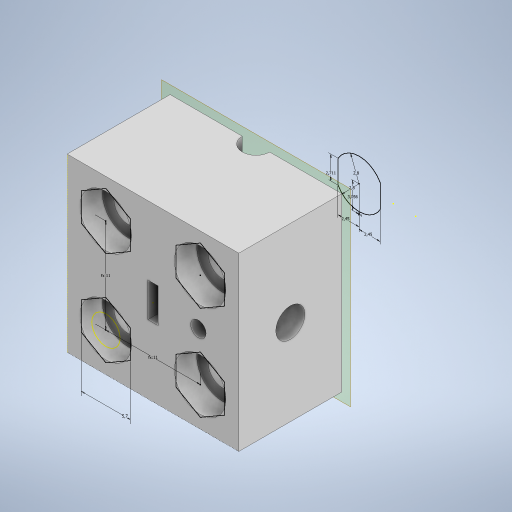
# Autodesk Inventor part: DFZ_bottom_fl_1mm_v3
Saved by Autodesk Inventor 2023 (Build 270158000, 158)
## iProperties
Created: 2019-07-31
Part Number: DFZ_bottom_fl_1mm_v3
Material: Generisch
Document SubType Name: Modeling
Designer: maximilian
Density: 1 g/cm^3
Appearance: Vorgabe
Author: maximilian
Autodesk Inventor part; units mm, degrees
ref_plane "YZ Plane" through (0, 0, 0) normal (1, 0, 0) x (0, 1, 0)
ref_plane "XZ Plane" through (0, 0, 0) normal (0, 1, 0) x (-1, 0, 0)
ref_plane "XY Plane" through (0, 0, 0) normal (0, 0, 1) x (1, 0, 0)
sketch "Skizze1" plane through (0, 0, 0) normal (0, 0, 1) x (1, 0, 0)
  line L0 (10, -10) -> (-10, -10)
  line L1 (-10, -10) -> (-10, 10)
  line L2 (-10, 10) -> (10, 10)
  line L3 (10, 10) -> (10, -10)
  line L4 (10, -10) -> (-10, 10) construction
  line L5 (-10, -10) -> (10, 10) construction
  point P0 (0, 0)
  dimension "d0" = 20
  dimension "d1" = 20
  constraints: 12 end point, 2 midpoint, 2 parallel, 1 horizontal, 1 perpendicular
  measures "d0" distance of L1.end L2.end
  measures "d1" distance of L0.end L1.end
extrude "Extrusion1" add sketch "Skizze1" along normal blind 24
sketch "Skizze2" plane through (-10, 10, 0) normal (0, 1, 0) x (1, 0, 0)
  line L0 (20, 0) -> (0, 0) construction
  line L1 (20, -24) -> (0, -24) construction
  line L2 (0, 0) -> (20, -24) construction
  line L3 (20, 0) -> (0, -24) construction
  circle A0 centre (10, -12) radius 1.6
  point P0 (10, 0)
  dimension "d4" = 3.2
  constraints: 4 end point, 1 centre point, 1 midpoint
  measures "d4" diameter of A0
extrude "Extrusion2" cut sketch "Skizze2" against normal through all
sketch "Skizze3" plane through (0, 0, 0) normal (0, 0, -1) x (-1, 0, 0)
  line L0 (-2.45, 1.3555) -> (-2.45, -1.3555)
  line L1 (2.45, -1.3555) -> (2.45, 1.3555)
  arc A0 (2.45, 1.3555) -> (-2.45, 1.3555) centre (0, 0) ccw
  arc A1 (-2.45, -1.3555) -> (2.45, -1.3555) centre (0, 0) ccw
  point P0 (0, -3.0564)
  dimension "d82" = 0
  dimension "d83" = 2.7111
  dimension "d84" = 2.8
  dimension "d85" = 2.8
  dimension "d86" = 2.45
  dimension "d87" = 2.45
  dimension "d88" = 3.0564
  constraints: 4 end point, 4 point on circle, 2 centre point, 1 coincident, 1 parallel
  measures "d82" horizontal distance of point (0, 0) point (0, -3.056)
  measures "d83" distance of L1.start L1.end
  measures "d84" radius of A1
  measures "d85" radius of A0
  measures "d86" distance from line of point (0, 0) L0
  measures "d87" horizontal distance of point (0, 0) L1.start
  measures "d88" distance of point (0, 0) point (0, -3.056)
extrude "Extrusion3" cut sketch "Skizze3" against normal through all
ref_plane "Arbeitsebene1" through (0, 0, 12) normal (0, 0, -1) x (-1, 0, 0)
sketch "Skizze4" plane through (0, 0, 0) normal (0, 0, -1) x (-1, 0, 0)
  line L0 (-10, -10) -> (-10, 10) projected
  line L1 (10, -10) -> (-10, -10) projected
  point P0 (0, 0)
  point P1 (-5.5, -5.5)
  point P2 (-5.5, 5.5)
  point P3 (5.5, -5.5)
  point P4 (5.5, 5.5)
  dimension "d11" = 4.5
  dimension "d12" = 4.5
  dimension "d15" = 11
  dimension "d18" = 11
  constraints: 1 horizontal, 1 vertical, 3 other
  measures "d11" distance from line of L0 point (-5.5, -5.5)
  measures "d12" distance from line of L1 point (-5.5, -5.5)
  measures "d15" distance of point (-5.5, -5.5) point (-5.5, 5.5)
  measures "d18" distance of point (-5.5, -5.5) point (5.5, -5.5)
hole "Bohrung1" at (5.5, -5.5, 0) at (5.5, 5.5, 0) at (-5.5, -5.5, 0) at (-5.5, 5.5, 0) direction (0, 0, 1) diameter 3.3 end through all counterbore diameter 5.5 counterbore depth 3.1
sketch "Skizze5" plane through (0, 0, 24) normal (0, 0, 1) x (1, 0, 0)
  circle A0 centre (-5.5, -5.5) radius 1.65 projected
  line L0 (-8.35, -3.8546) -> (-5.5, -2.2091)
  line L1 (-5.5, -2.2091) -> (-2.65, -3.8546)
  line L2 (-2.65, -3.8546) -> (-2.65, -7.1454)
  line L3 (-2.65, -7.1454) -> (-5.5, -8.7909)
  line L4 (-5.5, -8.7909) -> (-8.35, -7.1454)
  line L5 (-8.35, -7.1454) -> (-8.35, -3.8546)
  line L6 (-10, 10) -> (-10, -10) construction
  line L7 (-10, -10) -> (10, -10) construction
  line L8 (-10, -10) -> (10, -10) construction
  line L9 (2.65, -3.8546) -> (5.5, -2.2091)
  line L10 (5.5, -2.2091) -> (8.35, -3.8546)
  line L11 (8.35, -3.8546) -> (8.35, -7.1454)
  line L12 (8.35, -7.1454) -> (5.5, -8.7909)
  line L13 (5.5, -8.7909) -> (2.65, -7.1454)
  line L14 (2.65, -7.1454) -> (2.65, -3.8546)
  line L15 (-8.35, 7.1454) -> (-5.5, 8.7909)
  line L16 (-5.5, 8.7909) -> (-2.65, 7.1454)
  line L17 (-2.65, 7.1454) -> (-2.65, 3.8546)
  line L18 (-2.65, 3.8546) -> (-5.5, 2.2091)
  line L19 (-5.5, 2.2091) -> (-8.35, 3.8546)
  line L20 (-8.35, 3.8546) -> (-8.35, 7.1454)
  line L21 (2.65, 7.1454) -> (5.5, 8.7909)
  line L22 (5.5, 8.7909) -> (8.35, 7.1454)
  line L23 (8.35, 7.1454) -> (8.35, 3.8546)
  line L24 (8.35, 3.8546) -> (5.5, 2.2091)
  line L25 (5.5, 2.2091) -> (2.65, 3.8546)
  line L26 (2.65, 3.8546) -> (2.65, 7.1454)
  point P0 (0, 0)
  point P1 (5.5, -5.5)
  point P2 (-5.5, 5.5)
  point P3 (5.5, 5.5)
  dimension "d28" = 5.7
  dimension "d31" = 11
  dimension "d34" = 11
  constraints: 50 end point, 2 vertical, 1 coincident, 1 collinear, 1 horizontal, 52 other
  measures "d28" distance between parallel lines of L2 L5
  measures "d31" distance of point (-5.5, -5.5) point (5.5, -5.5)
  measures "d34" distance of point (-5.5, -5.5) point (-5.5, 5.5)
sketch "Skizze6" plane through (10, -10, 0) normal (1, 0, 0) x (0, 0, -1)
  line L0 (-10.4, 0) -> (-13.6, 0) construction
  line L1 (-24, 0) -> (-24, 20) construction
  line L2 (-12, 0) -> (-24, 20) construction
  line L3 (0, 20) -> (-24, 20) construction
  line L4 (0, 0) -> (-24, 0) construction
  line L5 (-12, 20) -> (-24, 0) construction
  line L6 (0, 20) -> (0, 0) construction
  line L7 (-12, 20) -> (0, 0) construction
  line L8 (0, 20) -> (-12, 0) construction
  point P0 (0, 10)
  point P1 (-18, 10)
  point P2 (-6, 10)
  constraints: 8 end point, 4 midpoint
hole "Bohrung2" at (10, 0, 18) at (10, 0, 6) direction (-1, 0, 0) diameter 2.5 depth 10 tip angle 118 counterbore diameter 5.9 counterbore depth 3.4125
split body "Trennen1" result two bodies by plane through (0, 0, 12) normal (0, 0, -1) first body at (-1.614, 9.39, 0.5)
ref_plane "Arbeitsebene2" through (-1.7063, 0, 18) normal (1, 0, 0) x (0, 0, -1)
ref_plane "Arbeitsebene3" through (-1.7063, 0, 18) normal (1, 0, 0) x (0, 0, -1)
sketch "Skizze7" plane through (6.5875, 0, 18) normal (1, 0, 0) x (0, 0, -1)
  line L0 (-57.5, 24.1046) -> (-60.35, 22.4591)
  line L1 (-57.5, 27.3954) -> (-57.5, 24.1046)
  line L2 (-60.35, 22.4591) -> (-63.2, 24.1046)
  line L3 (-60.35, 29.0409) -> (-57.5, 27.3954)
  circle A0 centre (-60.35, 25.75) radius 1.7
  line L4 (-63.2, 24.1046) -> (-63.2, 27.3954)
  line L5 (-63.2, 27.3954) -> (-60.35, 29.0409)
  line L6 (-60.35, 22.4591) -> (-45.6, 22.4591)
  line L7 (-60.35, 29.0409) -> (-45.6, 29.0409)
  line L8 (-45.6, 22.4591) -> (-45.6, 29.0409)
  line L9 (-57.5, 24.1046) -> (-60.35, 22.4591)
  line L10 (-57.5, 27.3954) -> (-57.5, 24.1046)
  line L11 (-60.35, 22.4591) -> (-63.2, 24.1046)
  line L12 (-60.35, 29.0409) -> (-57.5, 27.3954)
  circle A1 centre (-60.35, 25.75) radius 1.7
  line L13 (-63.2, 24.1046) -> (-63.2, 27.3954)
  line L14 (-63.2, 27.3954) -> (-60.35, 29.0409)
  line L15 (-60.35, 22.4591) -> (-45.6, 22.4591)
  line L16 (-60.35, 29.0409) -> (-45.6, 29.0409)
  line L17 (-45.6, 22.4591) -> (-45.6, 29.0409)
  circle A2 centre (0, 0) radius 1.25 projected
  line L18 (2.85, -1.6454) -> (0, -3.2909)
  line L19 (2.85, 1.6454) -> (2.85, -1.6454)
  circle A3 centre (0, 0) radius 1.7
  line L20 (0, 3.2909) -> (2.85, 1.6454)
  line L21 (-2.85, -1.6454) -> (-2.85, 1.6454)
  line L22 (-2.85, 1.6454) -> (0, 3.2909)
  line L23 (0, 3.2909) -> (14.75, 3.2909)
  line L24 (14.75, -3.2909) -> (14.75, 3.2909)
  line L25 (0, -3.2909) -> (14.75, -3.2909)
  line L26 (0, -3.2909) -> (-2.85, -1.6454)
  line L27 (2.85, -1.6454) -> (0, -3.2909)
  line L28 (2.85, 1.6454) -> (2.85, -1.6454)
  circle A4 centre (0, 0) radius 1.7
  line L29 (0, 3.2909) -> (2.85, 1.6454)
  line L30 (-2.85, -1.6454) -> (-2.85, 1.6454)
  line L31 (-2.85, 1.6454) -> (0, 3.2909)
  line L32 (0, 3.2909) -> (14.75, 3.2909)
  line L33 (14.75, -3.2909) -> (14.75, 3.2909)
  line L34 (0, -3.2909) -> (14.75, -3.2909)
  line L35 (0, -3.2909) -> (-2.85, -1.6454)
  point P0 (18, 0)
  dimension "d46" = 5.7
  dimension "d47" = 5.7
  dimension "d48" = 5.7
  dimension "d49" = 5.7
  constraints: 72 end point, 5 coincident, 4 centre point, 52 other
  measures "d46" distance between parallel lines of L4 L1
  measures "d47" distance between parallel lines of L13 L10
  measures "d48" distance between parallel lines of L21 L19
  measures "d49" distance between parallel lines of L30 L28
extrude "Extrusion5" cut sketch "Skizze7" against normal blind 2.6 contours L19 L20 L23 L24 L25 L18 | L18 L26 L21 L22 L20 L19 bodies 3
sketch "Skizze9" plane through (6.5875, 0, 18) normal (1, 0, 0) x (0, 0, -1)
  circle A0 centre (0, 0) radius 1.25
  circle A1 centre (0, 0) radius 2.95
  point P0 (18, 0)
  constraints: 2 centre point, 1 coincident
sketch "Skizze10" plane through (6.5875, 0, 18) normal (1, 0, 0) x (0, 0, -1)
  circle A0 centre (0, 0) radius 1.25 projected
  circle A1 centre (0, 0) radius 1.7
  point P0 (18, 0)
  constraints: 1 centre point, 1 coincident
extrude "Extrusion6" cut sketch "Skizze10" against normal up to surface (2.6 mm away) bodies 3
sketch "Skizze11" plane through (3.9875, 0, 18) normal (1, 0, 0) x (0, 0, -1)
  point P0 (18, 0)
sketch "Skizze12" plane through (10, 10, 12) normal (0, 0, -1) x (-1, 0, 0)
  line L0 (0, -20) -> (0, 0) projected
  line L1 (0, -13.2909) -> (0, -6.6893)
  line L2 (3.4125, -6.6893) -> (3.4125, -13.2909)
  line L3 (3.4125, -8.3546) -> (6.0125, -8.3546) projected
  line L4 (6.0125, -8.3546) -> (0, -8.3546)
  line L5 (0, -12.95) -> (0, -7.05) projected
  line L6 (3.4125, -11.6454) -> (6.0125, -11.6454) projected
  line L7 (6.0125, -11.6454) -> (0, -11.6454)
  point P0 (10, -10)
  point P1 (0, -11.6454)
  point P2 (0, -8.3546)
  constraints: 8 end point, 3 point on line, 2 perpendicular, 1 parallel
extrude "Extrusion7" add sketch "Skizze12" against normal up to surface (12 mm away) bodies 3
sketch "Skizze13" plane through (10, -10, 24) normal (1, 0, 0) x (0, 0, -1)
  circle A0 centre (6, 10) radius 1.25 projected
  circle A1 centre (6, 10) radius 1.25
  circle A2 centre (6, 10) radius 1.7
  point P0 (24, 10)
  dimension "d72" = 2.5
  dimension "d73" = 3.4
  constraints: 2 centre point, 2 coincident
  measures "d72" diameter of A0
  measures "d73" diameter of A2
extrude "Extrusion8" cut sketch "Skizze13" against normal blind 5 contours A0 bodies 3
sketch "Skizze14" plane through (10, -10, 24) normal (1, 0, 0) x (0, 0, -1)
  circle A0 centre (6, 10) radius 1.25 projected
  circle A1 centre (6, 10) radius 2.95
  line L0 (8.4485, 8.3546) -> (3.5515, 8.3546) projected
  line L1 (3.5515, 8.3546) -> (8.4485, 8.3546)
  arc A2 (8.4485, 11.6454) -> (5.2345, 12.849) centre (6, 10) ccw projected
  line L2 (3.5515, 11.6454) -> (8.4485, 11.6454)
  point P0 (24, 10)
  constraints: 5 end point, 2 point on circle, 1 centre point, 1 coincident, 1 collinear, 1 horizontal
extrude "Extrusion9" add sketch "Skizze14" against normal up to surface (3.4125 mm away) contours L2 A1 | A1 L0 bodies 3
sketch "Skizze15" plane through (10, -10, 12) normal (0, 0, -1) x (-1, 0, 0)
  line L0 (6.0125, 6.7091) -> (6.0125, 8.3546) construction
  line L1 (3.4125, 13.2909) -> (3.4125, 11.6454) construction
  line L2 (6.0125, 6.7091) -> (3.4125, 13.2909) construction
  line L3 (3.4125, 8.3546) -> (3.4125, 6.7091) construction
  line L4 (3.4125, 13.2909) -> (3.4125, 6.7091) construction
  line L5 (6.0125, 11.6454) -> (6.0125, 13.2909) construction
  line L6 (3.4125, 6.7091) -> (6.0125, 13.2909) construction
  circle A0 centre (4.7125, 10) radius 0.9
  point P0 (10, 10)
  dimension "d63" = 1.8
  constraints: 6 end point, 1 centre point, 1 collinear, 1 midpoint
  measures "d63" diameter of A0
extrude "Extrusion10" cut sketch "Skizze15" against normal through all bodies 3
sketch "Skizze16" plane through (0, 0, 24) normal (0, 0, 1) x (1, 0, 0)
  circle A0 centre (-5.5, 5.5) radius 1.65 projected
  circle A1 centre (-5.5, 5.5) radius 3
  circle A2 centre (5.5, 5.5) radius 1.65 projected
  circle A3 centre (5.5, 5.5) radius 3
  circle A4 centre (5.5, -5.5) radius 1.65 projected
  circle A5 centre (5.5, -5.5) radius 3
  circle A6 centre (-5.5, -5.5) radius 1.65 projected
  circle A7 centre (-5.5, -5.5) radius 3
  point P0 (0, 0)
  dimension "d66" = 6
  dimension "d67" = 6
  dimension "d68" = 6
  dimension "d69" = 6
  constraints: 4 centre point, 4 coincident
  measures "d66" diameter of A1
  measures "d67" diameter of A3
  measures "d68" diameter of A7
  measures "d69" diameter of A5
extrude "Extrusion11" cut sketch "Skizze16" against normal blind 2.6 bodies 3
sketch "Skizze17" plane through (10, -10, 24) normal (1, 0, 0) x (0, 0, -1)
  circle A0 centre (6, 10) radius 1.25 projected
  circle A1 centre (6, 10) radius 1.7
  point P0 (24, 10)
  dimension "d74" = 3.4
  constraints: 1 centre point, 1 coincident
  measures "d74" diameter of A1
extrude "Extrusion12" cut sketch "Skizze17" against normal blind 10 contours A0 | A1 bodies 3
sketch "Skizze18" plane through (-10, -10, 24) normal (-1, 0, 0) x (0, 0, 1)
  line L0 (-12, 0) -> (-12, 12.2978) construction
  line L1 (-12, 20) -> (0, 20) construction
  line L2 (-12, 0) -> (0, 20) construction
  line L3 (0, 20) -> (-12, 20) construction
  line L4 (-12, 0) -> (0, 0) construction
  line L5 (-12, 20) -> (0, 0) construction
  line L6 (-6, 10) -> (-12, 10) construction
  line L7 (-12, 12.2978) -> (-12, 12.2978) construction
  circle A0 centre (-12, 10) radius 1.8
  point P0 (-24, 10)
  dimension "d77" = 3.6
  constraints: 8 end point, 1 centre point, 1 coincident, 1 collinear, 1 midpoint, 1 point on line
  measures "d77" diameter of A0
extrude "Extrusion13" cut sketch "Skizze18" against normal blind 10 bodies 3
sketch "Skizze19" plane through (0, 0, 24) normal (0, 0, 1) x (1, 0, 0)
  line L0 (2.45, -1.3555) -> (2.45, 1.3555)
  line L1 (-2.45, 1.3555) -> (-2.45, -1.3555)
  line L2 (-0.6, -2) -> (0.6, -2)
  line L3 (0.6, -2) -> (0.6, 2)
  line L4 (0.6, 2) -> (-0.6, 2)
  line L5 (-0.6, 2) -> (-0.6, -2)
  arc A0 (-2.45, -1.3555) -> (2.45, -1.3555) centre (0, 0) ccw
  arc A1 (2.45, 1.3555) -> (-2.45, 1.3555) centre (0, 0) ccw
  point P0 (0, 0)
  point P1 (0, 3.114)
  dimension "d93" = 1.2
  dimension "d94" = 4
  dimension "d95" = 0.6
  dimension "d96" = 2
  dimension "d99" = 0
  dimension "d100" = 2.45
  dimension "d101" = 2.8
  dimension "d102" = 2.8
  dimension "d103" = 2.45
  dimension "d104" = 3.114
  dimension "d105" = 2.45
  constraints: 12 end point, 4 point on circle, 3 parallel, 2 centre point, 1 coincident, 1 horizontal, 1 perpendicular
  measures "d93" distance of L4.end L3.end
  measures "d94" distance of L3.end L2.end
  measures "d95" distance from line of point (0, 0) L3
  measures "d96" distance from line of point (0, 0) L4
  measures "d99" horizontal distance of point (0, 0) point (0, 3.114)
  measures "d100" distance from line of point (0, 0) L0
  measures "d101" radius of A1
  measures "d102" radius of A0
  measures "d103" horizontal distance of point (0, 0) L1.end
  measures "d104" distance of point (0, 0) point (0, 3.114)
  measures "d105" horizontal distance of point (0, 0) L0.start
extrude "Extrusion14" add sketch "Skizze19" against normal blind 6 bodies 3
equation "\"d15\" = d1 - 2 * d12"
equation "\"d18\" = d1 - 2 * d12"
equation "\"d31\" = d1 - 2 * d12"
equation "\"d34\" = d1 - 2 * d12"
equation "\"d95\" = 0.5 * d93"
equation "\"d96\" = 0.5 * d94"
equation "\"d10\" = -0.5 * d2"
equation "\"d2\" = 24"
